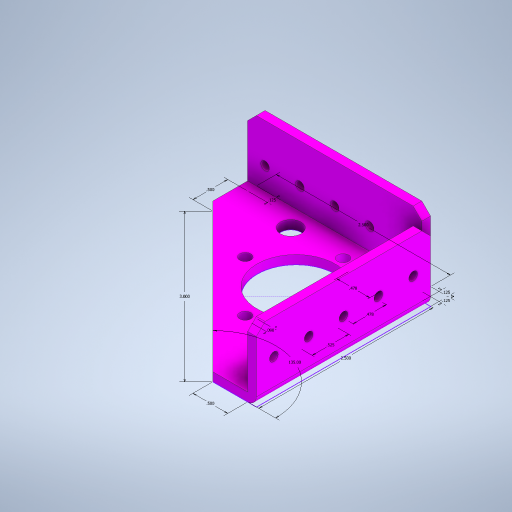
# Autodesk Inventor part: triangular L-bracket
Saved by Autodesk Inventor 2023 (Build 270158030, 158C)
## iProperties
Created: 2022-07-22
Part Number: triangular L-bracket
Material: Generic
Document SubType Name: Modeling
Designer: kt1040502
Density: 1 g/cm^3
Appearance: Default
Author: kt1040502
Autodesk Inventor part; units mm, degrees
ref_plane "YZ Plane" through (0, 0, 0) normal (1, 0, 0) x (0, 1, 0)
ref_plane "XZ Plane" through (0, 0, 0) normal (0, 1, 0) x (-1, 0, 0)
ref_plane "XY Plane" through (0, 0, 0) normal (0, 0, 1) x (1, 0, 0)
sketch "Sketch1" plane through (0, 0, 0) normal (0, 1, 0) x (-1, 0, 0)
  line L0 (0, 0) -> (0, -63.5)
  line L1 (0, -63.5) -> (3.175, -63.5)
  line L2 (3.175, -63.5) -> (3.175, 0)
  line L3 (3.175, 0) -> (0, 0)
  line L4 (3.175, 0) -> (15.875, 0)
  line L5 (15.875, 0) -> (69.7565, -53.8815)
  line L6 (69.7565, -53.8815) -> (69.7565, -66.5815)
  line L7 (69.7565, -66.5815) -> (69.7565, -69.7565)
  line L8 (69.7565, -69.7565) -> (6.2565, -69.7565)
  line L9 (6.2565, -69.7565) -> (6.2565, -66.5815)
  line L10 (6.2565, -66.5815) -> (69.7565, -66.5815)
  arc A0 (6.2565, -66.5815) -> (3.175, -63.5) centre (4.7158, -65.0408) ccw
  circle A1 centre (10.1629, -59.5936) radius 3.6195
  line L11 (10.1629, -55.9741) -> (10.1629, -43.8456) construction
  circle A2 centre (10.1629, -41.8136) radius 2.032
  line L12 (13.7824, -59.5936) -> (25.9236, -59.5936) construction
  circle A3 centre (27.9556, -59.5936) radius 2.032
  line L13 (6.2565, -63.5) -> (42.8158, -26.9408) construction
  circle A4 centre (27.6295, -42.127) radius 14.224
  circle A5 centre (46.1715, -42.127) radius 2.032
  line L14 (27.6295, -27.903) -> (27.6295, -25.617) construction
  circle A6 centre (27.6295, -23.585) radius 2.032
  circle A7 centre (47.0691, -59.5936) radius 3.7465
  line L15 (10.1629, -39.7816) -> (10.1629, -26.4466) construction
  circle A8 centre (10.1629, -22.7001) radius 3.7465
  dimension "d6" = 63.5
  dimension "d7" = 3.175
  dimension "d8" = 12.7
  dimension "d9" = 76.2
  dimension "d10" = 135
  dimension "d11" = 12.7
  dimension "d12" = 3.175
  dimension "d13" = 63.5
  dimension "d14" = 3.175
  dimension "d18" = 12.1285
  dimension "d20" = 12.1412
  dimension "d26" = 2.286
  dimension "d30" = 13.335
  constraints: 32 end point, 7 point on circle, 6 centre point, 6 perpendicular, 4 vertical, 3 vertical alignment, 2 point on line, 1 horizontal, 1 midpoint, 6 other
  measures "d6" distance of L0.start L0.end
  measures "d7" distance of L0.end L1.end
  measures "d8" distance of L2.end L4.end
  measures "d9" distance of L4.end L5.end
  measures "d10" angle of L4 L5
  measures "d11" distance of L5.end L6.end
  measures "d12" distance of L6.end L7.end
  measures "d13" distance of L7.end L8.end
  measures "d14" distance of L8.end L9.end
  measures "d18" distance of L11.start L11.end
  measures "d20" distance of L12.start L12.end
  measures "d26" distance of L14.start L14.end
  measures "d30" distance of L15.start L15.end
extrude "Extrusion1" add sketch "Sketch1" along normal blind 3.175 contours L4 L5 L6 L10 A0 L2
extrude "Extrusion2" add sketch "Sketch1" along normal blind 25.4 contours L3 L2 L1 L0 | L10 L7 L8 L9
chamfer "Chamfer1" distance 3.175 angle 45 4 edges at (-6.2565, 25.4, -68.169) (-1.5875, 25.4, -63.5) (-1.5875, 25.4, 0) (-69.7565, 25.4, -68.169)
sketch "Sketch2" plane through (0, 0, 0) normal (1, 0, 0) x (0, 0, -1)
  line L0 (0, 3.175) -> (0, 22.225) projected
  circle A0 centre (6.35, 12.7) radius 1.5875
  circle A1 centre (19.05, 12.7) radius 1.5875
  circle A2 centre (31.75, 12.7) radius 1.5875
  circle A3 centre (44.45, 12.7) radius 1.5875
  circle A4 centre (57.15, 12.7) radius 1.5875
  point P0 (0, 0)
  dimension "d44" = 3.175
  dimension "d46" = 3.175
  dimension "d48" = 3.175
  dimension "d50" = 3.175
  constraints: 5 centre point
  measures "d44" diameter of A1
  measures "d46" diameter of A2
  measures "d48" diameter of A3
  measures "d50" diameter of A4
sketch "Sketch3" plane through (-6.2565, 0, -69.7565) normal (0, 0, -1) x (-1, 0, 0)
  line L0 (0, 0) -> (0, 22.225) projected
  circle A0 centre (6.35, 11.1125) radius 1.5875
  circle A1 centre (19.05, 11.1125) radius 1.5875
  circle A2 centre (31.75, 11.1125) radius 1.5875
  circle A3 centre (44.45, 11.1125) radius 1.5875
  circle A4 centre (57.15, 11.1125) radius 1.5875
  point P0 (-6.2565, 0)
  dimension "d54" = 3.175
  dimension "d56" = 3.175
  dimension "d58" = 3.175
  dimension "d60" = 3.175
  dimension "d62" = 3.175
  constraints: 5 centre point
  measures "d54" diameter of A0
  measures "d56" diameter of A1
  measures "d58" diameter of A2
  measures "d60" diameter of A3
  measures "d62" diameter of A4
extrude "Extrusion3" cut sketch "Sketch2" against normal blind 3.175
extrude "Extrusion4" cut sketch "Sketch3" against normal blind 3.175
fillet "Fillet1" radius 3.175 2 edges at (0, 0, -31.75) (-38.0065, 0, -69.7565)
body "Solid1"
